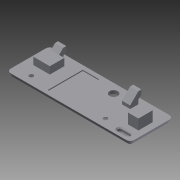
# Autodesk Inventor part: cap2
Saved by Autodesk Inventor 2014 SP2 (Build 180246200, 246)
## iProperties
Created: 2025-01-13
Part Number: cap2
Material: Generic
Document SubType Name: Sheet Metal
Designer: GauchoHP
Density: 1 g/cm^3
Sheet Metal Rule: Default_mm
Appearance: Default
Author: GauchoHP
Autodesk Inventor part; units mm, degrees
ref_plane "YZ Plane" through (0, 0, 0) normal (1, 0, 0) x (0, 1, 0)
ref_plane "XZ Plane" through (0, 0, 0) normal (0, 1, 0) x (-1, 0, 0)
ref_plane "XY Plane" through (0, 0, 0) normal (0, 0, 1) x (1, 0, 0)
sketch "Sketch1" plane through (0, 0, 0) normal (0, 0, 1) x (1, 0, 0)
  line L0 (-13.9727, 7.4707) -> (42.0273, 7.4707)
  line L1 (44.0273, 5.4707) -> (44.0273, -11.5293)
  line L2 (42.0273, -13.5293) -> (-13.9727, -13.5293)
  line L3 (-15.9727, -11.5293) -> (-15.9727, 5.4707)
  arc A0 (-13.9727, 7.4707) -> (-15.9727, 5.4707) centre (-13.9727, 5.4707) ccw
  arc A1 (-15.9727, -11.5293) -> (-13.9727, -13.5293) centre (-13.9727, -11.5293) ccw
  arc A2 (42.0273, -13.5293) -> (44.0273, -11.5293) centre (42.0273, -11.5293) ccw
  arc A3 (44.0273, 5.4707) -> (42.0273, 7.4707) centre (42.0273, 5.4707) ccw
  point P0 (0, 0)
  point P1 (44.0273, -13.5293)
  point P2 (44.0273, 7.4707)
  point P3 (-15.9727, -13.5293)
  dimension "d0" = 60
  dimension "d1" = 21
  dimension "d2" = 2
  dimension "d3" = 2
  constraints: 8 end point, 8 point on circle, 8 tangent, 6 point on line, 4 centre point, 2 equal radius, 2 parallel, 1 horizontal, 1 perpendicular
  measures "d0" distance of point (44.027, -13.529) point (-15.973, -13.529)
  measures "d1" distance of point (44.027, 7.471) point (44.027, -13.529)
  measures "d2" radius of A0
  measures "d3" radius of A1
extrude "Extrusion1" add sketch "Sketch1" along normal blind 2
chamfer "Chamfer1" distance 1 distance2 2 8 edges at (14.0273, -13.5293, 0) (-15.3869, -12.9435, 0) (-15.9727, -3.0293, 0) (-15.3869, 6.8849, 0) (14.0273, 7.4707, 0) (43.4415, 6.8849, 0) (44.0273, -3.0293, 0) (43.4415, -12.9435, 0) measured on face at (43.088, -12.59, 0) measured on face at (14.0273, -13.0293, 0) measured on face at (43.5273, -3.0293, 0) measured on face at (-15.0333, -12.59, 0) measured on face at (43.088, 6.5313, 0) measured on face at (14.0273, 6.9707, 0) measured on face at (-15.0333, 6.5313, 0) measured on face at (-15.4727, -3.0293, 0)
sketch "Sketch2" plane through (0, 0, 2) normal (0, 0, 1) x (1, 0, 0)
  line L0 (-13.9727, -13.5293) -> (42.0273, -13.5293) projected
  line L1 (44.0273, -11.5293) -> (44.0273, 5.4707) projected
  circle A0 centre (28.0273, -9.5293) radius 1
  circle A1 centre (-7.9727, -9.5293) radius 1
  point P0 (0, 0)
  dimension "d9" = 2
  dimension "d10" = 4
  dimension "d11" = 16
  dimension "d12" = 2
  dimension "d13" = 36
  constraints: 2 centre point
  measures "d9" diameter of A0
  measures "d10" distance from line of L0 A0.centre
  measures "d11" distance from line of L1 A0.centre
  measures "d12" diameter of A1
  measures "d13" distance between centres of A0 A1
extrude "Extrusion2" cut sketch "Sketch2" against normal blind 2
chamfer "Chamfer2" distance 2 angle 45 2 edges at (27.0273, -9.5293, 0) (-8.9727, -9.5293, 0)
sketch "Sketch3" plane through (0, 0, 2) normal (0, 0, 1) x (1, 0, 0)
  line L0 (42.0273, 7.4707) -> (-13.9727, 7.4707) projected
  line L1 (-15.9727, 5.4707) -> (-15.9727, -11.5293) projected
  line L2 (44.0273, -11.5293) -> (44.0273, 5.4707) projected
  line L3 (30.0273, 0.4707) -> (26.0273, 0.4707)
  line L4 (26.0273, 0.4707) -> (26.0273, 4.4707)
  line L5 (26.0273, 4.4707) -> (30.0273, 4.4707)
  line L6 (30.0273, 4.4707) -> (30.0273, 0.4707)
  line L7 (-6.4727, 0.4707) -> (-10.4727, 0.4707)
  line L8 (-10.4727, 0.4707) -> (-10.4727, 4.4707)
  line L9 (-10.4727, 4.4707) -> (-6.4727, 4.4707)
  line L10 (-6.4727, 4.4707) -> (-6.4727, 0.4707)
  point P0 (0, 0)
  dimension "d19" = 4
  dimension "d20" = 14
  dimension "d22" = 4
  dimension "d24" = 4
  dimension "d25" = 4
  dimension "d26" = 5.5
  dimension "d27" = 3
  dimension "d86" = 3
  constraints: 16 end point, 4 parallel, 2 horizontal, 2 perpendicular
  measures "d19" distance of L4.end L5.end
  measures "d20" distance between parallel lines of L2 L6
  measures "d22" distance of L5.end L3.start
  measures "d24" distance of L8.end L9.end
  measures "d25" distance of L7.end L8.end
  measures "d26" distance between parallel lines of L8 L1
  measures "d27" distance between parallel lines of L0 L9
  measures "d86" distance between parallel lines of L0 L5
extrude "Extrusion3" add sketch "Sketch3" along normal blind 5.5
sketch "Sketch4" plane through (26.0273, 4.4707, 2) normal (0, 1, 0) x (1, 0, 0)
  line L0 (4, 0) -> (4, -5.5) projected
  line L1 (0, -5.5) -> (4, -5.5)
  line L2 (4, -5.5) -> (4, -3.5)
  line L3 (4, -3.5) -> (0, -3.5)
  line L4 (0, -3.5) -> (0, -5.5)
  point P0 (-26.0273, 2)
  dimension "d30" = 2
  constraints: 8 end point, 2 parallel, 1 horizontal, 1 perpendicular, 1 point on line
  measures "d30" distance of L2.end L1.end
extrude "Extrusion4" add sketch "Sketch4" along normal blind 1.5
chamfer "Chamfer3" distance 1.5 angle 45 1 edges at (28.0273, 4.4707, 5.5)
sketch "Sketch5" plane through (-10.4727, 4.4707, 2) normal (0, 1, 0) x (1, 0, 0)
  line L0 (4, 0) -> (4, -5.5) projected
  line L1 (0, -5.5) -> (4, -5.5)
  line L2 (4, -5.5) -> (4, -3.5)
  line L3 (4, -3.5) -> (0, -3.5)
  line L4 (0, -3.5) -> (0, -5.5)
  point P0 (10.4727, 2)
  dimension "d36" = 2
  constraints: 8 end point, 2 parallel, 1 horizontal, 1 perpendicular, 1 point on line
  measures "d36" distance of L2.end L1.end
extrude "Extrusion5" add sketch "Sketch5" along normal blind 1.5
chamfer "Chamfer4" distance 1.5 angle 45 1 edges at (-8.4727, 4.4707, 5.5)
chamfer "Chamfer5" distance 4 angle 45 2 edges at (-8.4727, 0.4707, 7.5) (28.0273, 0.4707, 7.5)
sketch "Sketch6" plane through (0, 0, 2) normal (0, 0, 1) x (1, 0, 0)
  line L0 (42.0273, 7.4707) -> (-13.9727, 7.4707) projected
  line L1 (-13.9727, -13.5293) -> (42.0273, -13.5293) projected
  line L2 (44.0273, -11.5293) -> (44.0273, 5.4707) projected
  line L3 (36.0273, 0.4707) -> (41.0273, 0.4707)
  line L4 (41.0273, 0.4707) -> (41.0273, -6.5293)
  line L5 (41.0273, -6.5293) -> (36.0273, -6.5293)
  line L6 (36.0273, -6.5293) -> (36.0273, 0.4707)
  point P0 (0, 0)
  dimension "d45" = 5
  dimension "d46" = 7
  dimension "d47" = 3
  dimension "d48" = 7
  dimension "d49" = 7
  constraints: 8 end point, 2 parallel, 1 horizontal, 1 perpendicular
  measures "d45" distance of L4.end L5.end
  measures "d46" distance of L3.end L4.end
  measures "d47" distance between parallel lines of L2 L4
  measures "d48" distance between parallel lines of L0 L3
  measures "d49" distance between parallel lines of L1 L5
extrude "Extrusion6" add sketch "Sketch6" along normal blind 5
sketch "Sketch7" plane through (0, 0, 2) normal (0, 0, 1) x (1, 0, 0)
  line L0 (42.0273, 7.4707) -> (-13.9727, 7.4707) projected
  line L1 (44.0273, -11.5293) -> (44.0273, 5.4707) projected
  line L2 (36.0273, 5.4707) -> (40.0273, 5.4707)
  line L3 (41.0273, 4.4707) -> (41.0273, 3.4707)
  line L4 (35.0273, 4.4707) -> (35.0273, 4.4707)
  line L5 (41.0273, -6.5293) -> (36.0273, -6.5293) projected
  line L6 (-13.9727, -13.5293) -> (42.0273, -13.5293) projected
  line L7 (36.0273, -9.5293) -> (40.0273, -9.5293)
  line L8 (41.0273, -10.5293) -> (41.0273, -10.5293)
  line L9 (40.0273, -11.5293) -> (36.0273, -11.5293)
  line L10 (35.0273, -10.5293) -> (35.0273, -10.5293)
  arc A0 (36.0273, 5.4707) -> (35.0273, 4.4707) centre (36.0273, 4.4707) ccw
  arc A1 (41.0273, 4.4707) -> (40.0273, 5.4707) centre (40.0273, 4.4707) ccw
  arc A2 (40.0273, 2.4707) -> (41.0273, 3.4707) centre (40.0273, 3.4707) ccw
  arc A3 (35.0273, 4.4707) -> (36.0273, 3.4707) centre (36.0273, 4.4707) ccw
  arc A4 (36.0273, -9.5293) -> (35.0273, -10.5293) centre (36.0273, -10.5293) ccw
  arc A5 (35.0273, -10.5293) -> (36.0273, -11.5293) centre (36.0273, -10.5293) ccw
  arc A6 (40.0273, -11.5293) -> (41.0273, -10.5293) centre (40.0273, -10.5293) ccw
  arc A7 (41.0273, -10.5293) -> (40.0273, -9.5293) centre (40.0273, -10.5293) ccw
  point P0 (0, 0)
  point P1 (35.0273, 5.4707)
  point P2 (41.0273, 3.4707)
  point P3 (41.0273, 5.4707)
  point P4 (35.0273, 3.4707)
  point P5 (41.0273, -11.5293)
  point P6 (41.0273, -9.5293)
  point P7 (35.0273, -11.5293)
  dimension "d52" = 6
  dimension "d53" = 2
  dimension "d54" = 3
  dimension "d55" = 2
  dimension "d58" = 6
  dimension "d59" = 2
  dimension "d60" = 3
  dimension "d61" = 2
  dimension "d62" = 3
  dimension "d64" = 1
  constraints: 16 point on circle, 14 end point, 14 tangent, 12 point on line, 8 centre point, 7 equal radius, 3 parallel, 2 horizontal, 2 perpendicular
  measures "d52" distance of point (41.027, 3.471) point (35.027, 3.471)
  measures "d53" distance of point (41.027, 5.471) point (41.027, 3.471)
  measures "d54" distance between parallel lines of L1 L3
  measures "d55" distance between parallel lines of L0 L2
  measures "d58" distance of point (41.027, -11.529) point (35.027, -11.529)
  measures "d59" distance of point (41.027, -9.529) point (41.027, -11.529)
  measures "d60" distance between parallel lines of L1 L8
  measures "d61" distance between parallel lines of L6 L9
  measures "d62" distance between parallel lines of L5 L7
  measures "d64" radius of A0
extrude "Extrusion7" cut sketch "Sketch7" against normal blind 10
chamfer "Chamfer6" distance 0.5 angle 45 8 edges at (38.0273, -11.5293, 2) (35.0273, -10.5293, 2) (38.0273, -9.5293, 2) (41.0273, -10.5293, 2) (38.0273, -9.5293, 0) (35.0273, -10.5293, 0) (38.0273, -11.5293, 0) (41.0273, -10.5293, 0)
sketch "Sketch8" plane through (0, 0, 2) normal (0, 0, 1) x (1, 0, 0)
  line L0 (44.0273, -11.5293) -> (44.0273, 5.4707) projected
  circle A0 centre (19.5273, 2.9707) radius 2
  line L1 (42.0273, 7.4707) -> (-13.9727, 7.4707) projected
  point P0 (0, 0)
  dimension "d68" = 4
  dimension "d69" = 24.5
  dimension "d76" = 4.5
  constraints: 1 centre point
  measures "d68" diameter of A0
  measures "d69" distance from line of L0 A0.centre
  measures "d76" distance from line of L1 A0.centre
extrude "Extrusion8" cut sketch "Sketch8" against normal blind 10
chamfer "Chamfer7" distance 0.5 angle 45 1 edges at (17.5273, 2.9707, 0)
sketch "Sketch9" plane through (0, 0, 2) normal (0, 0, 1) x (1, 0, 0)
  line L0 (-15.9727, 5.4707) -> (-15.9727, -11.5293) projected
  line L1 (-13.9727, -13.5293) -> (42.0273, -13.5293) projected
  line L2 (-11.9727, 2.4707) -> (-3.9727, 2.4707)
  line L3 (-3.9727, 2.4707) -> (-3.9727, -4.5293)
  line L4 (-3.9727, -4.5293) -> (-11.9727, -4.5293)
  line L5 (-11.9727, -4.5293) -> (-11.9727, 2.4707)
  point P0 (0, 0)
  dimension "d77" = 8
  dimension "d78" = 7
  dimension "d81" = 4
  dimension "d87" = 9
  constraints: 8 end point, 2 parallel, 1 horizontal, 1 perpendicular
  measures "d77" distance of L3.end L4.end
  measures "d78" distance of L2.end L3.end
  measures "d81" distance between parallel lines of L0 L5
  measures "d87" distance between parallel lines of L4 L1
extrude "Extrusion9" add sketch "Sketch9" along normal blind 3.5
sketch "Sketch10" plane through (0, 0, 2) normal (0, 0, 1) x (1, 0, 0)
  line L0 (42.0273, 7.4707) -> (-13.9727, 7.4707) projected
  line L1 (-13.9727, -13.5293) -> (42.0273, -13.5293) projected
  line L2 (44.0273, -11.5293) -> (44.0273, 5.4707) projected
  line L3 (2.0273, 5.4707) -> (10.0273, 5.4707)
  line L4 (10.0273, 5.4707) -> (10.0273, -11.5293)
  line L5 (10.0273, -11.5293) -> (2.0273, -11.5293)
  line L6 (2.0273, -11.5293) -> (2.0273, 5.4707)
  point P0 (0, 0)
  dimension "d88" = 34
  dimension "d89" = 8
  dimension "d90" = 2
  dimension "d91" = 2
  constraints: 8 end point, 2 parallel, 1 horizontal, 1 perpendicular
  measures "d88" distance between parallel lines of L2 L4
  measures "d89" distance of L4.end L5.end
  measures "d90" distance between parallel lines of L1 L5
  measures "d91" distance between parallel lines of L0 L3
extrude "Extrusion10" cut sketch "Sketch10" against normal blind 0.5
equation "\"BendRadius\" = Thickness"
equation "\"BendReliefWidth\" = Thickness"
equation "\"BendReliefDepth\" = 0.5 * Thickness"
equation "\"CornerReliefSize\" = 4 * Thickness"
equation "\"MinimumRemnant\" = 2 * Thickness"
equation "\"TransitionRadius\" = BendRadius"
equation "\"JacobiRadiusSize\" = BendRadius"
equation "\"GapSize\" = Thickness"
equation "\"Thickness\" = 0.5"
body "Solid1"
